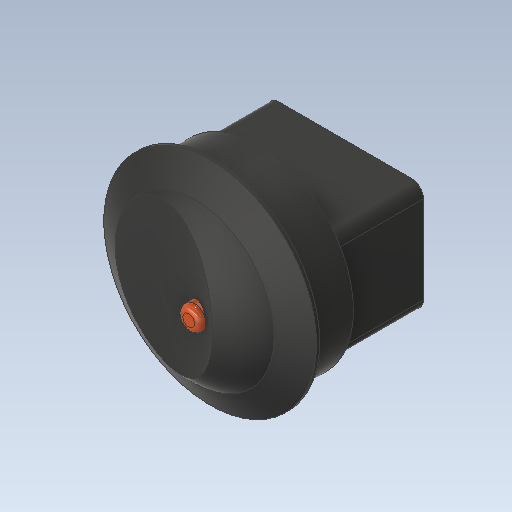
# Autodesk Inventor part: Power Switch
Saved by Autodesk Inventor 2020 (Build 240168000, 168)
## iProperties
Created: 2019-01-12
Part Number: Power Switch
Material: Generic
Document SubType Name: Modeling
Designer: LSabe
Density: 1 g/cm^3
Appearance: Default
Author: LSabe
Autodesk Inventor part; units mm, degrees
ref_plane "YZ Plane" through (0, 0, 0) normal (1, 0, 0) x (0, 1, 0)
ref_plane "XZ Plane" through (0, 0, 0) normal (0, 1, 0) x (-1, 0, 0)
ref_plane "XY Plane" through (0, 0, 0) normal (0, 0, 1) x (1, 0, 0)
sketch "Sketch1" plane through (0, 0, 0) normal (0, 0, 1) x (1, 0, 0)
  circle A0 centre (0, 0) radius 10.414
  dimension "d0" = 20.828
  constraints: 1 centre point, 1 coincident
  measures "d0" diameter of A0
extrude "Extrusion1" add sketch "Sketch1" along normal blind 4.826
sketch "Sketch2" plane through (0, 0, 4.826) normal (0, 0, 1) x (1, 0, 0)
  circle A0 centre (0, 0) radius 11.557
  dimension "d3" = 23.114
  constraints: 1 centre point, 1 coincident
  measures "d3" diameter of A0
extrude "Extrusion2" add sketch "Sketch2" along normal blind 2.032
chamfer "Chamfer1" distance 2.921 angle 30 1 edges at (-11.557, 0, 6.858) measured on face at (-11.057, 0, 6.858)
sketch "Sketch3" plane through (0, 0, 6.858) normal (0, 0, 1) x (1, 0, 0)
  circle A0 centre (0, 0) radius 8.636 projected
extrude "Extrusion3" add sketch "Sketch3" along normal blind 3.683
sketch "Sketch4" plane through (0, 0, 0) normal (0, 1, 0) x (-1, 0, 0)
  line L0 (-6.8437, 10.3572) -> (-8.636, 6.858)
  arc A0 (-6.5088, 10.4709) -> (8.636, 6.858) centre (9.5932, 44.419) ccw
  line L1 (8.636, 10.541) -> (-8.636, 10.541) projected
  line L2 (8.636, 6.858) -> (8.636, 10.541)
  line L3 (8.636, 6.858) -> (8.636, 10.541) projected
  line L4 (8.636, 10.541) -> (-8.636, 10.541)
  arc A1 (-6.5088, 10.4709) -> (-6.8437, 10.3572) centre (-6.6176, 10.2414) ccw
  line L5 (-8.636, 6.858) -> (-8.636, 10.541)
  point P0 (0, 0)
  point P1 (-6.731, 10.5772)
  dimension "d14" = 0.254
  constraints: 8 end point, 5 point on circle, 2 centre point, 2 tangent, 1 collinear, 1 perpendicular, 1 point on line, 1 vertical
  measures "d14" radius of A1
extrude "Extrusion4" cut sketch "Sketch4" along normal mid plane 25.4
sketch "Sketch5" plane through (0, 0, 0) normal (0, 1, 0) x (-1, 0, 0)
  line L0 (-8.636, 10.5319) -> (-1.1317, 10.5319)
  arc A0 (-1.1317, 10.5319) -> (-8.636, 6.858) centre (-0.3466, -0.5729) ccw
  line L1 (-8.636, 6.858) -> (-8.636, 10.5319)
  line L2 (0, -2.94) -> (0, 13.6297) projected
  point P0 (0, 0)
  constraints: 4 end point, 2 point on circle, 1 centre point
revolve "Revolution1" cut sketch "Sketch5" angle 360 about axis through (0, 0, -10) along (0, 0, 1)
sketch "Sketch6" plane through (0, 0, 0) normal (0, 0, -1) x (-1, 0, 0)
  line L0 (-8.4836, -6.0325) -> (8.4836, -6.0325)
  line L1 (8.4836, -6.0325) -> (8.4836, 6.0325)
  line L2 (8.4836, 6.0325) -> (-8.4836, 6.0325)
  line L3 (-8.4836, 6.0325) -> (-8.4836, -6.0325)
  line L4 (-8.4836, -6.0325) -> (8.4836, 6.0325) construction
  line L5 (8.4836, -6.0325) -> (-8.4836, 6.0325) construction
  point P0 (0, 0)
  dimension "d21" = 16.9672
  dimension "d22" = 12.065
  constraints: 12 end point, 2 midpoint, 2 parallel, 1 horizontal, 1 perpendicular
  measures "d21" distance of L2.end L1.end
  measures "d22" distance of L1.end L0.end
extrude "Extrusion5" add sketch "Sketch6" along normal blind 9.525
fillet "Fillet1" radius 1.27 4 edges at (8.4836, 6.0325, -4.7625) (-8.4836, 6.0325, -4.7625) (-8.4836, -6.0325, -4.7625) (8.4836, -6.0325, -4.7625)
sketch "Sketch7" plane through (0, 0, -9.525) normal (0, 0, -1) x (-1, 0, 0)
  point P0 (0, 0)
sketch "Sketch8" plane through (0, 0, 4.826) normal (0, 0, -1) x (-1, 0, 0)
  circle A0 centre (-2.3902, 0) radius 1.27
  point P0 (0, 0)
  dimension "d26" = 2.54
  constraints: 1 centre point
  measures "d26" diameter of A0
extrude "Extrusion6" add sketch "Sketch8" against normal blind 5.08
fillet "Fillet2" radius 0.635 1 edges at (3.6602, 0, 9.906)
body "Solid1"
